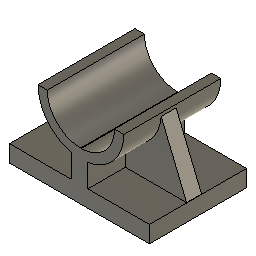
Practice Model 1 (Autodesk Fusion 360 design; units mm, degrees)
part number: 2026-05-21-16-34-07-399
Autodesk Fusion 360 part; units mm, degrees
note: some values were not read from the file. Set by a fixed rule: which sketch regions a step uses.
sketch "Sketch1" plane through (0, 0, 0) normal (0, 0, 1) x (1, 0, 0)
  line L0 (-66.176, 27.9285) -> (8.824, 27.9285)
  line L1 (8.824, 27.9285) -> (8.824, -24.0715)
  line L2 (8.824, -24.0715) -> (-66.176, -24.0715)
  line L3 (-66.176, -24.0715) -> (-66.176, 27.9285)
  dimension "d1" = 75
  dimension "d2" = 52
  constraint horizontal L0
  constraint vertical L1
  constraint horizontal L2
  constraint vertical L3
  measures "d1" distance of L0.start L0.end
  measures "d2" distance of L0.start L2.end
extrude "Extrude1" add sketch "Sketch1" along normal blind 9
sketch "Sketch2" plane through (0, 0, 9) normal (0, 0, 1) x (-1, 0, 0)
  line L0 (66.176, 24.0715) -> (-8.824, 24.0715)
  line L1 (-8.824, 24.0715) -> (-8.824, -27.9285)
  line L2 (-8.824, -27.9285) -> (66.176, -27.9285)
  line L3 (66.176, -27.9285) -> (66.176, 24.0715)
  line L4 (33.176, -27.9285) -> (24.176, -27.9285)
  line L5 (24.176, -27.9285) -> (24.176, 24.0715)
  line L6 (24.176, 24.0715) -> (33.176, 24.0715)
  line L7 (33.176, 24.0715) -> (33.176, -27.9285)
  line L8 (24.176, 24.0715) -> (-8.824, 24.0715)
  dimension "d5" = 9
  dimension "d6" = 52
  dimension "d7" = 33
  constraint horizontal L4
  constraint vertical L5
  constraint horizontal L6
  constraint vertical L7
  constraint coincident L2 L4.start
  constraint coincident L0.end L1.start
  measures "d5" distance of L4.start L4.end
  measures "d6" distance of L4.start L6.end
  measures "d7" distance of L5.end L0.end
extrude "Extrude2" add sketch "Sketch2" along normal blind 17 contours L0 L2 L4 L5 L6 L7
sketch "Sketch4" plane through (0, -24.0715, 0) normal (0, -1, 0) x (1, 0, 0)
  line L0 (-66.176, 0) -> (8.824, 0)
  line L1 (8.824, 0) -> (8.824, 9)
  line L2 (8.824, 9) -> (-24.176, 9)
  line L3 (-24.176, 9) -> (-24.176, 26)
  line L4 (-24.176, 26) -> (-33.176, 26)
  line L5 (-33.176, 26) -> (-33.176, 9)
  line L6 (-33.176, 9) -> (-66.176, 9)
  line L7 (-66.176, 9) -> (-66.176, 0)
  line L8 (-9.8869, 43.9299) -> (-4.8869, 43.9108)
  line L9 (-45.8867, 43.9989) -> (-50.8867, 44.018)
  arc A0 (-45.8867, 43.9989) -> (-9.8869, 43.9299) centre (-27.8867, 43.9989) ccw
  arc A1 (-50.8867, 44.018) -> (-4.8869, 43.9108) centre (-27.8867, 43.9989) ccw
  dimension "d11" = 46
  dimension "d12" = 36
  constraint concentric A0 A1
  measures "d11" diameter of A1
  measures "d12" diameter of A0
extrude "Extrude3" add sketch "Sketch4" against normal blind 52 contours L4 L5 L9 A0 A1 | L3 L4 L5 A1 | L3 L4 L8 A0 A1
sketch "Sketch7" plane through (0, 0, 0) normal (0, 1, 0) x (1, 0, 0)
  line L0 (-5.3043, -43.059) -> (8.7257, -8.8004)
rib "Rib1" add thickness 8 on both sides direction (-0.925403, 0, -0.378983) up to next extending the curves path "Sketch7" along L0
